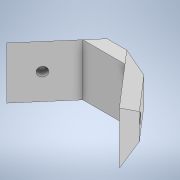
# Autodesk Inventor part: sun3
Saved by Autodesk Inventor 2021 (Build 250183000, 183)
## iProperties
Created: 2021-04-13
Part Number: sun3
Material: 일반
Document SubType Name: Modeling
Designer: Dongyoon
Density: 1 g/cm^3
Appearance: 기본값
Author: Dongyoon
Autodesk Inventor part; units mm, degrees
ref_plane "YZ Plane" through (0, 0, 0) normal (1, 0, 0) x (0, 1, 0)
ref_plane "XZ Plane" through (0, 0, 0) normal (0, 1, 0) x (-1, 0, 0)
ref_plane "XY Plane" through (0, 0, 0) normal (0, 0, 1) x (1, 0, 0)
sketch "스케치1" plane through (0, 0, 0) normal (0, 1, 0) x (-1, 0, 0)
  line L0 (0, 0) -> (-8.1, 0)
  line L1 (-8.1, 0) -> (-21.65, 15.7)
  line L2 (-21.65, 15.7) -> (-21.65, 8.0474)
  line L3 (-21.65, 8.0474) -> (-10.3894, -5)
  line L4 (-10.3894, -5) -> (0, -5)
  line L5 (0, -5) -> (0, 0)
  line L6 (0, 0) -> (8.1, 0)
  line L7 (8.1, 0) -> (21.65, 15.7)
  line L8 (21.65, 15.7) -> (21.65, 8.0474)
  line L9 (21.65, 8.0474) -> (10.3894, -5)
  line L10 (10.3894, -5) -> (0, -5)
  dimension "d0" = 15.7
  dimension "d1" = 43.3
  dimension "d2" = 16.2
  dimension "d3" = 5
  dimension "d4" = 5
  constraints: 22 end point, 4 symmetric about line, 2 parallel, 1 horizontal, 1 perpendicular, 1 vertical
  measures "d0" distance from line of L1.end L0
  measures "d1" distance between parallel lines of L8 L2
  measures "d2" distance of L6.end L0.end
  measures "d3" distance between parallel lines of L3 L1
  measures "d4" distance between parallel lines of L0 L4
extrude "돌출1" add sketch "스케치1" along normal blind 20
sketch "스케치2" plane through (21.65, 0, 15.7) normal (-0.7570398, 0, 0.6533688) x (0.6533688, 0, 0.7570398)
  line L0 (-20.7387, 20) -> (0, 20) projected
  line L1 (-9.7387, 20) -> (-9.7387, 0)
  line L2 (-20.7387, 0) -> (0, 0) projected
  line L3 (0, 0) -> (0, 20) projected
  line L4 (-20.7387, 0) -> (-20.7387, 20) projected
  circle A0 centre (-9.7387, 10) radius 1.75
  point P0 (-26.031, 0)
  dimension "d8" = 11
  dimension "d9" = 3.5
  dimension "d10" = 10
  dimension "d11" = 11
  constraints: 2 end point, 2 point on line, 1 centre point, 1 vertical
  measures "d8" distance between parallel lines of L4 L1
  measures "d9" diameter of A0
  measures "d10" distance from line of L0 A0.centre
  measures "d11" distance from line of L4 A0.centre
extrude "돌출2" cut sketch "스케치2" against normal through all contours A0 L1 | L1 A0
mirror "미러1" about plane through (0, 0, 0) normal (1, 0, 0) of "돌출2"
chamfer "모따기1" distance 5 angle 45 4 edges at (16.0197, 20, 1.5237) (-16.0197, 20, 1.5237) (16.0197, 0, 1.5237) (-16.0197, 0, 1.5237)
